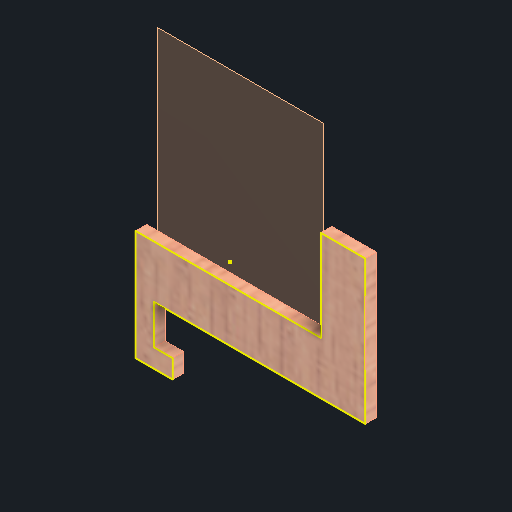
# Autodesk Inventor part: Button Bracket 1
Saved by Autodesk Inventor 2025.2 (Build 292293000, 293)
## iProperties
Created: 2024-11-20
Part Number: Button Bracket 1
Material: Wood (Oak)
Document SubType Name: Modeling
Designer: JL
Density: 0.76 g/cm^3
Appearance: White Oak - Natural Medium Gloss
Author: JL
Autodesk Inventor part; units mm, degrees
ref_plane "YZ Plane" through (0, 0, 0) normal (1, 0, 0) x (0, 1, 0)
ref_plane "XZ Plane" through (0, 0, 0) normal (0, 1, 0) x (-1, 0, 0)
ref_plane "XY Plane" through (0, 0, 0) normal (0, 0, 1) x (1, 0, 0)
ref_plane "Work Plane1" through (0, 0, 0) normal (0, 0, 1) x (1, 0, 0)
sketch "Sketch1" plane through (0, 0, 0) normal (0, 0, 1) x (1, 0, 0)
  line L0 (10, -5.5) -> (10, 39) construction
  line L1 (-10, 39) -> (10, 39) construction
  line L2 (-10, -5.5) -> (-10, 39) construction
  line L3 (-20.35, -5.5) -> (-10, -5.5) projected
  line L4 (-20.35, -19.6) -> (-20.35, -5.5) projected
  line L5 (20.35, -19.6) -> (-20.35, -19.6) projected
  line L6 (20.35, -19.6) -> (20.35, -5.5) projected
  line L7 (10, -5.5) -> (20.35, -5.5) projected
  line L8 (-20.35, -30.2) -> (-20.35, 45.6) projected
  line L9 (20.35, -30.2) -> (-20.35, -30.2) projected
  line L10 (-10, -5.5) -> (10, -5.5)
  line L11 (-20.35, -5.5) -> (-25.35, -5.5)
  line L12 (-25.35, -5.5) -> (-25.35, -35.2)
  line L13 (-25.35, -35.2) -> (-15.35, -35.2)
  line L14 (-15.35, -35.2) -> (-15.35, -30.2)
  line L15 (20.35, -19.6) -> (36.5729, -19.6)
  line L16 (36.5729, -19.6) -> (36.5729, 19)
  line L17 (36.5729, 19) -> (24.5729, 19)
  line L18 (24.5729, 19) -> (24.5729, -5.5)
  line L19 (24.5729, -5.5) -> (20.35, -5.5)
  line L20 (36.5729, 7) -> (24.5729, 7) construction
  line L21 (24.5729, 7) -> (24.5729, 19) construction
  line L22 (24.5729, 19) -> (36.5729, 19) construction
  line L23 (36.5729, 19) -> (36.5729, 7) construction
  point P0 (0, 0)
  dimension "d0" = 5
  dimension "d1" = 5
  dimension "d2" = 5
  constraints: 20 end point, 7 perpendicular, 2 horizontal, 1 point on line, 1 vertical
  measures "d0" distance of L3.start L11.end
  measures "d1" distance of L13.end L14.end
  measures "d2" distance from line of L8.start L14
extrude "Extrusion1" add sketch "Sketch1" along normal blind 3
sketch "Sketch2" plane through (0, 0, 3) normal (0, 0, 1) x (1, 0, 0)
  line L0 (-15.35, -35.2) -> (-15.35, -30.2) projected
  line L1 (-15.35, -30.2) -> (-20.35, -30.2) projected
  line L2 (-20.35, -30.2) -> (-20.35, -19.6) projected
  line L3 (-20.35, -19.6) -> (36.5729, -19.6) projected
  line L4 (36.5729, -19.6) -> (36.5729, 19) projected
  line L5 (36.5729, 19) -> (24.5729, 19) projected
  line L6 (24.5729, 19) -> (24.5729, -5.5) projected
  line L7 (24.5729, -5.5) -> (-25.35, -5.5) projected
  line L8 (-25.35, -5.5) -> (-25.35, -35.2) projected
  line L9 (-25.35, -35.2) -> (-15.35, -35.2) projected
  point P0 (0, 0)
equation "\"d1\" = d0"
equation "\"d2\" = d0"
body "Solid1"
